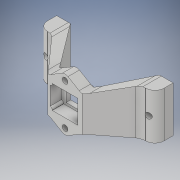
# Autodesk Inventor part: еще 1 новое крепление потенциометра
Saved by Autodesk Inventor 2019.1 (Build 231200000, 200)
## iProperties
Created: 2018-09-16
Part Number: еще 1 новое крепление потенциометра
Material: Типовые
Document SubType Name: Modeling
Designer: Олег
Density: 1 g/cm^3
Appearance: По умолчанию
Author: Олег
Autodesk Inventor part; units mm, degrees
ref_plane "YZ Plane" through (0, 0, 0) normal (1, 0, 0) x (0, 1, 0)
ref_plane "XZ Plane" through (0, 0, 0) normal (0, 1, 0) x (-1, 0, 0)
sketch "Эскиз1" plane through (0, 0, 0) normal (0, 0, 1) x (1, 0, 0)
  circle A0 centre (-22.5, 0) radius 1.25
  circle A1 centre (22.5, 0) radius 1.25
  line L0 (-19.5, -10) -> (-25.5, -10)
  line L1 (-25.5, -10) -> (-25.5, 10)
  line L2 (-25.5, 10) -> (-19.5, 10)
  line L3 (-19.5, 10) -> (-19.5, -10)
  line L4 (-19.5, -10) -> (-25.5, 10) construction
  line L5 (-25.5, -10) -> (-19.5, 10) construction
  line L6 (25.5, -10) -> (19.5, -10)
  line L7 (19.5, -10) -> (19.5, 10)
  line L8 (19.5, 10) -> (25.5, 10)
  line L9 (25.5, 10) -> (25.5, -10)
  line L10 (25.5, -10) -> (19.5, 10) construction
  line L11 (19.5, -10) -> (25.5, 10) construction
  point P0 (0, 0)
  dimension "d0" = 2.5
  dimension "d1" = 2.5
  dimension "d2" = 45
  dimension "d3" = 22.5
  dimension "d4" = 6
  dimension "d5" = 20
  dimension "d6" = 6
  dimension "d7" = 20
  constraints: 24 end point, 4 midpoint, 4 parallel, 2 centre point, 2 horizontal, 2 horizontal alignment, 2 perpendicular
  measures "d0" diameter of A0
  measures "d1" diameter of A1
  measures "d2" distance of A0.centre A1.centre
  measures "d3" distance of A0.centre point (0, 0)
  measures "d4" distance of L1.end L2.end
  measures "d5" distance of L0.end L1.end
  measures "d6" distance of L7.end L8.end
  measures "d7" distance of L6.end L7.end
extrude "Выдавливание1" add sketch "Эскиз1" along normal blind 8
ref_plane "РабПлоскость1" through (0, 0, 21.8) normal (0, 0, -1) x (-1, 0, 0)
sketch "Эскиз2" plane through (0, 0, 21.8) normal (0, 0, -1) x (-1, 0, 0)
  line L0 (-7.5, -7.5) -> (7.5, -7.5)
  line L1 (7.5, -7.5) -> (7.5, 7.5)
  line L2 (7.5, 7.5) -> (-7.5, 7.5)
  line L3 (-7.5, 7.5) -> (-7.5, -7.5)
  line L4 (-7.5, -7.5) -> (7.5, 7.5) construction
  line L5 (7.5, -7.5) -> (-7.5, 7.5) construction
  line L6 (5.6, -5.1) -> (-5.6, -5.1)
  line L7 (-5.6, -5.1) -> (-5.6, 5.1)
  line L8 (-5.6, 5.1) -> (5.6, 5.1)
  line L9 (5.6, 5.1) -> (5.6, -5.1)
  line L10 (5.6, -5.1) -> (-5.6, 5.1) construction
  line L11 (-5.6, -5.1) -> (5.6, 5.1) construction
  point P0 (0, 0)
  dimension "d11" = 15
  dimension "d12" = 15
  dimension "d43" = 11.2
  dimension "d44" = 10.2
  constraints: 24 end point, 4 midpoint, 4 parallel, 2 horizontal, 2 perpendicular
  measures "d11" distance of L2.end L1.end
  measures "d12" distance of L1.end L0.end
  measures "d43" distance of L7.end L8.end
  measures "d44" distance of L6.end L7.end
extrude "Выдавливание7" add sketch "Эскиз2" along normal blind 5
loft "Лофт1" add section 1 edges at (-19.5, 0, 0) (-19.5, 10, 4) (-19.5, 0, 8) (-19.5, -10, 4) section 2 edges at (-7.5, 0, 21.8) (-7.5, 7.5, 19.3) (-7.5, 0, 16.8) (-7.5, -7.5, 19.3)
loft "Лофт2" add section 1 edges at (19.5, 0, 0) (19.5, -10, 4) (19.5, 0, 8) (19.5, 10, 4) section 2 edges at (7.5, 0, 21.8) (7.5, -7.5, 19.3) (7.5, 0, 16.8) (7.5, 7.5, 19.3)
sketch "Эскиз7" plane through (0, 0, 16.8) normal (0, 0, -1) x (-1, 0, 0)
  line L0 (5.6, 5.1) -> (5.6, -5.1) projected
  line L1 (-4.6, 5.1) -> (4.6, 5.1)
  line L2 (5.6, 4.1) -> (5.6, -4.1)
  line L3 (4.6, -5.1) -> (-4.6, -5.1)
  line L4 (-5.6, -4.1) -> (-5.6, 4.1)
  line L5 (-5.6, 5.1) -> (5.6, -5.1) construction
  line L6 (5.6, 5.1) -> (-5.6, -5.1) construction
  arc A0 (4.6, -5.1) -> (5.6, -4.1) centre (4.6, -4.1) ccw
  arc A1 (-5.6, -4.1) -> (-4.6, -5.1) centre (-4.6, -4.1) ccw
  arc A2 (-4.6, 5.1) -> (-5.6, 4.1) centre (-4.6, 4.1) ccw
  arc A3 (5.6, 4.1) -> (4.6, 5.1) centre (4.6, 4.1) ccw
  line L7 (-4.6, -6.1) -> (4.6, -6.1)
  arc A4 (4.6, -6.1) -> (6.6, -4.1) centre (4.6, -4.1) ccw
  line L8 (6.6, -4.1) -> (6.6, 4.1)
  arc A5 (6.6, 4.1) -> (4.6, 6.1) centre (4.6, 4.1) ccw
  line L9 (4.6, 6.1) -> (-4.6, 6.1)
  arc A6 (-4.6, 6.1) -> (-6.6, 4.1) centre (-4.6, 4.1) ccw
  line L10 (-6.6, 4.1) -> (-6.6, -4.1)
  arc A7 (-6.6, -4.1) -> (-4.6, -6.1) centre (-4.6, -4.1) ccw
  line L11 (-4.6, -4.1) -> (4.6, -4.1)
  line L12 (4.6, -4.1) -> (4.6, 4.1)
  line L13 (4.6, 4.1) -> (-4.6, 4.1)
  line L14 (-4.6, 4.1) -> (-4.6, -4.1)
  point P0 (0, 0)
  dimension "d58" = 11.2
  dimension "d59" = 10.2
  dimension "d60" = 1
  dimension "d61" = 1
  dimension "d62" = 1
  constraints: 28 end point, 16 point on circle, 8 centre point, 8 point on line, 8 tangent, 6 parallel, 3 equal radius, 3 perpendicular, 2 midpoint, 1 horizontal, 10 other
  measures "d58" distance of L0.end L6.end
  measures "d59" distance of L6.start L0.end
  measures "d60" radius of A0
  measures "d61" distance between parallel lines of L3 L7
  measures "d62" distance between parallel lines of L3 L11
extrude "Выдавливание8" add sketch "Эскиз7" along normal blind 2 contours L0 A0 L3 A1 L4 A2 L1 A3 | A7 L10 A6 L9 A5 L8 A4 L7
sketch "Эскиз8" plane through (0, 0, 21.8) normal (0, 0, 1) x (1, 0, 0)
  line L0 (-4.6, -4) -> (-6.6, -4)
  line L1 (-6.6, -4) -> (-6.6, 4)
  line L2 (-6.6, 4) -> (-4.6, 4)
  line L3 (-4.6, 4) -> (-4.6, -4)
  line L4 (-5.6, 5.1) -> (-5.6, -5.1) projected
  line L5 (-4.6, -4) -> (-6.6, 4) construction
  line L6 (-6.6, -4) -> (-4.6, 4) construction
  point P0 (0, 0)
  point P1 (-5.6, 0)
  dimension "d66" = 2
  dimension "d67" = 8
  constraints: 12 end point, 3 midpoint, 2 parallel, 1 horizontal, 1 perpendicular
  measures "d66" distance of L1.end L2.end
  measures "d67" distance of L0.end L1.end
extrude "Выдавливание9" cut sketch "Эскиз8" against normal blind 5
fillet "Сопряжение3" radius 4 2 edges at (-19.5, 0, 8) (19.5, 0, 8)
fillet "Сопряжение4" radius 8 4 edges at (19.5, 10, 4) (-19.5, 10, 4) (-19.5, -10, 4) (19.5, -10, 4)
fillet "Сопряжение5" radius 4 2 edges at (-25.5, 0, 8) (25.5, 0, 8)
sketch "Эскиз10" plane through (0, 0, 21.8) normal (0, 0, 1) x (1, 0, 0)
  line L0 (-18.3041, 9.7509) -> (-7.5, 7.5) projected
  line L1 (-7.5, 7.5) -> (7.5, 7.5) projected
  line L2 (-7.5, 7.5) -> (7.5, 7.5)
  circle A0 centre (0, 9) radius 1.25
  line L3 (-7.5, 7.5) -> (-1.2646, 11.1565)
  line L4 (7.5, 7.5) -> (1.2646, 11.1565)
  arc A1 (1.2646, 11.1565) -> (-1.2646, 11.1565) centre (0, 9) ccw
  line L5 (0, 0) -> (0.71, 0) construction
  line L6 (-7.5, -7.5) -> (7.5, -7.5)
  circle A2 centre (0, -9) radius 1.25
  line L7 (-7.5, -7.5) -> (-1.2646, -11.1565)
  line L8 (7.5, -7.5) -> (1.2646, -11.1565)
  arc A3 (-1.2646, -11.1565) -> (1.2646, -11.1565) centre (0, -9) ccw
  dimension "d77" = 2.5
  dimension "d79" = 1.5
  dimension "d80" = 2.5
  constraints: 14 end point, 6 symmetric about line, 4 centre point, 4 point on circle, 2 coincident, 2 horizontal, 2 tangent, 1 vertical alignment, 2 other
  measures "d77" diameter of A0
  measures "d79" distance from line of L1 A0.centre
  measures "d80" radius of A1
extrude "Выдавливание11" add sketch "Эскиз10" against normal blind 5
fillet "Сопряжение12" radius 4 4 edges at (-7.5, -7.5, 19.3) (7.5, -7.5, 19.3) (7.5, 7.5, 19.3) (-7.5, 7.5, 19.3)
fillet "Сопряжение13" radius 1 2 edges at (-5.6, 4, 19.3) (-5.6, -4, 19.3)
equation "\"d3\" = 0.5 * d2"
